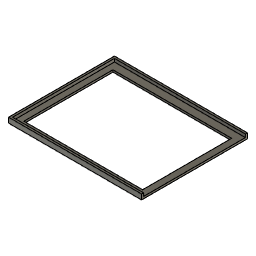
FrontPanel (Autodesk Fusion 360 design; units mm, degrees)
Autodesk Fusion 360 part; units mm, degrees
sketch "Sketch2" plane through (0, 0, 0) normal (0, 0, 1) x (1, 0, 0)
  line L0 (-55.8718, 52.373) -> (70.1282, 52.373)
  line L1 (70.1282, 52.373) -> (70.1282, -47.127)
  line L2 (70.1282, -47.127) -> (-55.8718, -47.127)
  line L3 (-55.8718, -47.127) -> (-55.8718, 52.373)
  line L4 (-50, 45) -> (66, 45)
  line L5 (66, 45) -> (66, -42)
  line L6 (66, -42) -> (-50, -42)
  line L7 (-50, -42) -> (-50, 45)
  line L8 (-57.8718, 54.373) -> (72.1282, 54.373)
  line L9 (72.1282, 54.373) -> (72.1282, -49.127)
  line L10 (72.1282, -49.127) -> (-57.8718, -49.127)
  line L11 (-57.8718, -49.127) -> (-57.8718, 54.373)
  dimension "d1" = 126
  dimension "d2" = 99.5
  dimension "d3" = 116
  dimension "d4" = 87
  dimension "d5" = 130
  dimension "d6" = 103.5
  dimension "d7" = 2
  dimension "d8" = 2
  constraint horizontal L0
  constraint vertical L1
  constraint horizontal L2
  constraint vertical L3
  constraint horizontal L4
  constraint vertical L5
  constraint horizontal L6
  constraint vertical L7
  constraint horizontal L8
  constraint vertical L9
  constraint horizontal L10
  constraint vertical L11
  measures "d1" distance of L0.start L0.end
  measures "d2" distance of L0.end L1.end
  measures "d3" distance of L4.start L4.end
  measures "d4" distance of L4.start L6.end
  measures "d5" distance of L8.start L8.end
  measures "d6" distance of L8.start L10.end
  measures "d7" distance of L0 L8
  measures "d8" distance of L3 L11
extrude "Extrude7" add sketch "Sketch2" along normal blind 2 contours L0 L1 L2 L3
extrude "Extrude8" add sketch "Sketch2" along normal blind 5 contours L8 L9 L10 L11
sketch "Sketch9" plane through (0, 0, 5) normal (0, 0, 1) x (-1, 0, 0)
  line L0 (-70.1282, 47.127) -> (55.8718, 47.127)
  line L1 (55.8718, 47.127) -> (55.8718, -52.373)
  line L2 (55.8718, -52.373) -> (-70.1282, -52.373)
  line L3 (-70.1282, -52.373) -> (-70.1282, 47.127)
  line L4 (57.8718, 49.127) -> (-72.1282, 49.127)
  line L5 (-72.1282, 49.127) -> (-72.1282, -54.373)
  line L6 (-72.1282, -54.373) -> (57.8718, -54.373)
  line L7 (57.8718, -54.373) -> (57.8718, 49.127)
  line L8 (-70.1282, -52.373) -> (-72.1282, -52.373)
  line L9 (-72.1282, -52.373) -> (-72.1282, 47.127)
  line L10 (-72.1282, 47.127) -> (-70.1282, 47.127)
  line L11 (-70.1282, 47.127) -> (-70.1282, -52.373)
  dimension "d39" = 99.5
  constraint horizontal L8
  constraint vertical L9
  constraint horizontal L10
  constraint vertical L11
  constraint coincident L5 L9.end
  constraint coincident L2.end L3.start
  measures "d39" distance of L8.end L9.end
extrude "Extrude9" cut sketch "Sketch9" against normal blind 3 contours L3 L5 L8 L9 L10 L11
